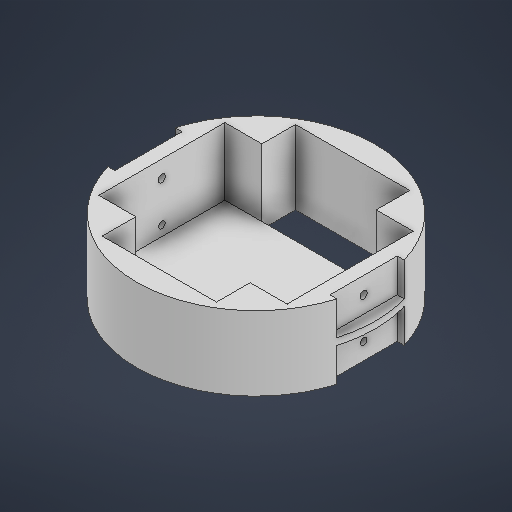
# Autodesk Inventor part: 002-002
Saved by Autodesk Inventor 2026 (Build 300175000, 175)
## iProperties
Created: 2026-04-19
Part Number: 002-002
Material: Ogólny
Document SubType Name: Modeling
Designer: Patryk Lombardo
Density: 1 g/cm^3
Appearance: Domyślna
Author: Patryk Lombardo
Autodesk Inventor part; units mm, degrees
ref_plane "YZ Plane" through (0, 0, 0) normal (1, 0, 0) x (0, 1, 0)
ref_plane "XZ Plane" through (0, 0, 0) normal (0, 1, 0) x (-1, 0, 0)
ref_plane "XY Plane" through (0, 0, 0) normal (0, 0, 1) x (1, 0, 0)
sketch "Szkic1" plane through (0, 0, 0) normal (0, 1, 0) x (-1, 0, 0)
  circle A0 centre (0, 0) radius 35.5
  line L0 (0, 18.75) -> (0, -18.75) construction
  line L1 (-28, 0) -> (28, 0) construction
  line L2 (-28, -18.75) -> (28, -18.75)
  line L3 (-28, 18.75) -> (-28, -18.75)
  line L4 (28, 18.75) -> (28, -18.75)
  line L5 (0, 18.75) -> (28, 18.75)
  line L6 (0, 18.75) -> (-28, 18.75)
  line L7 (0, 18.75) -> (0, 28.75) construction
  line L8 (17, 28.75) -> (-17, 28.75)
  line L9 (17, 28.75) -> (17, 18.75)
  line L10 (-17, 28.75) -> (-17, 18.75)
  line L11 (0, -18.75) -> (0, -28.75) construction
  line L12 (-17, -28.75) -> (17, -28.75)
  line L13 (17, -28.75) -> (17, -18.75)
  line L14 (-17, -28.75) -> (-17, -18.75)
  dimension "d0" = 71
  dimension "d1" = 37.5
  dimension "d2" = 56
  dimension "d4" = 10
  dimension "d5" = 34
  dimension "d16" = 10
  dimension "d17" = 34
  constraints: 30 end point, 7 midpoint, 5 horizontal, 5 vertical, 4 point on line, 3 perpendicular, 1 centre point, 1 coincident, 1 collinear
  measures "d0" diameter of A0
  measures "d1" distance of L0.start L0.end
  measures "d2" distance of L1.start L1.end
  measures "d4" distance of L0.start L7.end
  measures "d5" distance of L8.start L8.end
  measures "d16" distance of L0.end L11.end
  measures "d17" distance of L12.start L12.end
extrude "Wyciągnięcie proste1" add sketch "Szkic1" along normal blind 20
extrude "Wyciągnięcie proste2" add sketch "Szkic1" against normal blind 2 contours A0 | L3 L6 L5 L4 L2
sketch "Szkic2" plane through (0, 20, 0) normal (0, 1, 0) x (1, 0, 0)
  line L0 (32, 0) -> (-32, 0) construction
  circle A0 centre (0, 0) radius 35.5
  line L1 (-32, -10) -> (-32, 10)
  line L2 (32, -10) -> (32, 10)
  line L3 (32, -10) -> (34.0624, -10)
  line L4 (32, 10) -> (34.0624, 10)
  line L5 (-32, -10) -> (-34.0624, -10)
  line L6 (-32, 10) -> (-34.0624, 10)
  dimension "d10" = 64
  dimension "d11" = 71
  dimension "d12" = 20
  dimension "d13" = 20
  constraints: 14 end point, 4 horizontal, 4 point on circle, 3 midpoint, 2 vertical, 1 centre point, 1 coincident, 1 parallel
  measures "d10" distance of L0.start L0.end
  measures "d11" diameter of A0
  measures "d12" distance of L1.start L1.end
  measures "d13" distance of L2.start L2.end
extrude "Wyciągnięcie proste3" cut sketch "Szkic2" against normal blind 10 contours A0 L3 L2 L4 | L6 L1 L5 A0
sketch "Szkic3" plane through (32, 20, 10) normal (1, 0, 0) x (0, 0, -1)
  line L0 (0, 0) -> (10, 0) construction
  line L1 (10, 0) -> (10, -5) construction
  circle A0 centre (10, -5) radius 1.1
  point P0 (10, -20)
  dimension "d18" = 10
  dimension "d19" = 20
  dimension "d20" = 20
  dimension "d21" = 5
  dimension "d22" = 2.2
  constraints: 4 end point, 1 centre point, 1 coincident, 1 horizontal, 1 vertical
  measures "d18" distance of L0.start L0.end
  measures "d19" distance from line of point (10, -20) L0
  measures "d20" distance of point (10, -20) L0.end
  measures "d21" distance of L0.end L1.end
  measures "d22" diameter of A0
extrude "Wyciągnięcie proste4" cut sketch "Szkic3" against normal through all
sketch "Szkic7" plane through (0, -2, 0) normal (0, -1, 0) x (1, 0, 0)
  line L0 (32, 0) -> (-32, 0) construction
  circle A0 centre (0, 0) radius 35.5
  line L1 (-32, -10) -> (-32, 10)
  line L2 (32, -10) -> (32, 10)
  line L3 (32, -10) -> (34.0624, -10)
  line L4 (32, 10) -> (34.0624, 10)
  line L5 (-32, -10) -> (-34.0624, -10)
  line L6 (-32, 10) -> (-34.0624, 10)
  dimension "d48" = 64
  dimension "d49" = 71
  dimension "d50" = 20
  dimension "d51" = 20
  constraints: 14 end point, 4 horizontal, 4 point on circle, 3 midpoint, 2 coincident, 2 vertical, 1 centre point, 1 parallel
  measures "d48" distance of L0.start L0.end
  measures "d49" diameter of A0
  measures "d50" distance of L1.start L1.end
  measures "d51" distance of L2.start L2.end
extrude "Wyciągnięcie proste8" cut sketch "Szkic7" against normal blind 10 contours A0 L3 L2 L4 | L6 L1 L5 A0
sketch "Szkic8" plane through (32, -2, 10) normal (1, 0, 0) x (0, 0, -1)
  line L0 (10, 2) -> (10, 5) construction
  circle A0 centre (10, 5) radius 1
  dimension "d54" = 3
  dimension "d55" = 2
  constraints: 2 end point, 1 centre point, 1 coincident, 1 vertical
  measures "d54" distance of L0.start L0.end
  measures "d55" diameter of A0
extrude "Wyciągnięcie proste9" cut sketch "Szkic8" against normal through all
